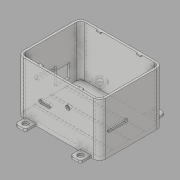
# Autodesk Inventor part: DispenserElectronicsBoxV2
Saved by Autodesk Inventor 2017 (Build 210142000, 142)
## iProperties
Created: 2017-05-31
Part Number: DispenserElectronicsBoxV2
Material: Generic
Document SubType Name: Modeling
Designer: gmarsh
Density: 1 g/cm^3
Appearance: Default
Author: gmarsh
Autodesk Inventor part; units mm, degrees
ref_plane "YZ Plane" through (0, 0, 0) normal (1, 0, 0) x (0, 1, 0)
ref_plane "XZ Plane" through (0, 0, 0) normal (0, 1, 0) x (-1, 0, 0)
ref_plane "XY Plane" through (0, 0, 0) normal (0, 0, 1) x (1, 0, 0)
sketch "Sketch1" plane through (0, 0, 0) normal (0, 0, 1) x (1, 0, 0)
  line L0 (-32.9996, 28) -> (32.9996, 28)
  line L1 (36.9996, 24) -> (36.9996, -24)
  line L2 (32.9996, -28) -> (-32.9996, -28)
  line L3 (-36.9996, -24) -> (-36.9996, 24)
  arc A0 (36.9996, 24) -> (32.9996, 28) centre (32.9996, 24) ccw
  arc A1 (32.9996, -28) -> (36.9996, -24) centre (32.9996, -24) ccw
  arc A2 (-36.9996, -24) -> (-32.9996, -28) centre (-32.9996, -24) ccw
  arc A3 (-32.9996, 28) -> (-36.9996, 24) centre (-32.9996, 24) ccw
  point P0 (0, 0)
  dimension "d0" = 4
  constraints: 8 end point, 8 point on circle, 8 tangent, 4 centre point, 3 equal radius, 2 parallel, 1 horizontal, 1 perpendicular
  measures "d0" radius of A0
surface extrude "ExtrusionSrf1" sketch "Sketch1" along normal blind 50 shown no curves L1 A1 L2 A2 L3 A3 L0 A0
thicken "Thicken1" operation new thickness 2 both sides no extend neighbours no toward (1, 0, 0) faces at (36.9996, 8, 16.6667) (35.7203, -26.9322, 33.3333) (10.9999, -28, 33.3333) (-35.7203, -26.9322, 33.3333) (-36.9996, -8, 16.6667) (-35.9318, 26.7207, 33.3333) (-10.9999, 28, 33.3333) (35.7203, 26.9322, 33.3333)
sketch "Sketch2" plane through (32.9996, -30, 0) normal (0, 0, -1) x (-1, 0, 0)
  line L0 (0, 58) -> (66.081, 58)
  line L1 (70.081, 54) -> (70.081, 6)
  line L2 (66.081, 2) -> (0, 2)
  line L3 (-4, 6) -> (-4, 54)
  arc A0 (70.081, 54) -> (66.081, 58) centre (66.081, 54) ccw
  arc A1 (66.081, 2) -> (70.081, 6) centre (66.081, 6) ccw
  arc A2 (-4, 6) -> (0, 2) centre (0, 6) ccw
  arc A3 (0, 58) -> (-4, 54) centre (0, 54) ccw
  point P0 (32.9996, 30)
  point P1 (31, 30)
  dimension "d5" = 4
  constraints: 8 end point, 8 point on circle, 8 tangent, 4 centre point, 3 equal radius, 2 parallel, 1 horizontal, 1 perpendicular
  measures "d5" radius of A0
extrude "Bottom" add sketch "Sketch2" against normal blind 2
sketch "Sketch9" plane through (32.9996, -30, 0) normal (0, 0, -1) x (-1, 0, 0)
  line L0 (61.976, 69.9481) -> (56.0348, 69.9481)
  line L1 (54.0348, 67.9481) -> (54.0348, -8.1004)
  line L2 (56.0348, -10.1004) -> (61.976, -10.1004)
  line L3 (63.976, -8.1004) -> (63.976, 67.9481)
  line L4 (4, -10.0079) -> (9.9992, -10.0079)
  line L5 (11.9992, -8.0079) -> (11.9992, 67.9122)
  line L6 (9.9992, 69.9122) -> (4, 69.9122)
  line L7 (2, 67.9122) -> (2, -8.0079)
  arc A0 (61.976, -10.1004) -> (63.976, -8.1004) centre (61.976, -8.1004) ccw
  arc A1 (54.0348, -8.1004) -> (56.0348, -10.1004) centre (56.0348, -8.1004) ccw
  arc A2 (63.976, 67.9481) -> (61.976, 69.9481) centre (61.976, 67.9481) ccw
  arc A3 (56.0348, 69.9481) -> (54.0348, 67.9481) centre (56.0348, 67.9481) ccw
  arc A4 (2, -8.0079) -> (4, -10.0079) centre (4, -8.0079) ccw
  arc A5 (9.9992, -10.0079) -> (11.9992, -8.0079) centre (9.9992, -8.0079) ccw
  arc A6 (11.9992, 67.9122) -> (9.9992, 69.9122) centre (9.9992, 67.9122) ccw
  arc A7 (4, 69.9122) -> (2, 67.9122) centre (4, 67.9122) ccw
  point P0 (32.9996, 30)
  point P1 (2, -10.0079)
  point P2 (11.9992, 69.9122)
  dimension "d18" = 2
  constraints: 16 end point, 16 point on circle, 16 tangent, 8 centre point, 7 equal radius, 4 parallel, 4 point on line, 2 horizontal, 2 perpendicular
  measures "d18" radius of A0
extrude "Mounting Tabs" add sketch "Sketch9" against normal blind 2
sketch "Sketch10" plane through (32.9996, -30, 2) normal (0, 0, 1) x (1, 0, 0)
  circle A0 centre (-59, 65) radius 2.5
  circle A1 centre (-7, 65) radius 2.5
  circle A2 centre (-7, -5) radius 2.5
  circle A3 centre (-59, -5) radius 2.5
  point P0 (-32.9996, 30)
  dimension "d21" = 5
  dimension "d22" = 5
  dimension "d23" = 5
  dimension "d24" = 5
  constraints: 4 centre point
  measures "d21" diameter of A0
  measures "d22" diameter of A1
  measures "d23" diameter of A2
  measures "d24" diameter of A3
extrude "Mounting Tab Holes" cut sketch "Sketch10" against normal blind 2
sketch "Sketch4" plane through (38.9996, -24, 0) normal (1, 0, 0) x (0, 0, -1)
  line L0 (-2, 48) -> (-2, 0) projected
  circle A0 centre (-2, 24) radius 1
  circle A1 centre (-2, 8) radius 1
  circle A2 centre (-2, 38) radius 1
  point P0 (0, 24)
  constraints: 3 centre point, 2 point on line, 1 midpoint
extrude "Bottom Ridges" add sketch "Sketch4" against normal blind 76
sketch "Sketch6" plane through (-32.9996, -28, 50) normal (0, 1, 0) x (1, 0, 0)
  line L0 (54, 0) -> (50, 0)
  line L1 (50, 0) -> (50, 1)
  line L2 (50, 1) -> (54, 1)
  line L3 (54, 1) -> (54, 0)
  line L4 (16, 0) -> (12, 0)
  line L5 (12, 0) -> (12, 1)
  line L6 (12, 1) -> (16, 1)
  line L7 (16, 1) -> (16, 0)
  point P0 (32.9996, 50)
  constraints: 16 end point, 4 parallel, 2 horizontal, 2 perpendicular, 2 point on line
extrude "Bottom Latch" add sketch "Sketch6" along normal blind 1
sketch "Sketch8" plane through (-32.9996, 28, 50) normal (0, -1, 0) x (1, 0, 0)
  line L0 (65.9992, 0) -> (0, 0) projected
  line L1 (12, -1) -> (16, -1) projected
  line L2 (12, 0) -> (16, 0)
  line L3 (16, 0) -> (16, -1)
  line L4 (16, -1) -> (12, -1)
  line L5 (12, -1) -> (12, 0)
  line L6 (50, -1) -> (50, 0) projected
  line L7 (54, -1) -> (50, -1) projected
  line L8 (50, 0) -> (54, 0)
  line L9 (54, 0) -> (54, -1)
  line L10 (54, -1) -> (50, -1)
  line L11 (50, -1) -> (50, 0)
  point P0 (32.9996, -50)
  constraints: 16 end point, 4 parallel, 2 horizontal, 2 perpendicular
extrude "Top Latch" add sketch "Sketch8" along normal blind 1
sketch "Sketch11" plane through (-38.9996, -24, 0) normal (-1, 0, 0) x (0, 0, 1)
  line L0 (22, 28) -> (22, 12) construction
  line L1 (20.5, 28) -> (20.5, 12)
  line L2 (23.5, 12) -> (23.5, 28)
  arc A0 (23.5, 28) -> (20.5, 28) centre (22, 28) ccw
  arc A1 (20.5, 12) -> (23.5, 12) centre (22, 12) ccw
  line L3 (20, 29) -> (7.0332, 29)
  line L4 (7.0332, 29) -> (7.0332, 41.9562)
  line L5 (7.0332, 41.9562) -> (20, 41.9562)
  line L6 (20, 41.9562) -> (20, 29)
  line L7 (8, 10) -> (20, 10)
  line L8 (20, 10) -> (20, 0)
  line L9 (20, 0) -> (8, 0)
  line L10 (8, 0) -> (8, 10)
  point P0 (0, 24)
  point P1 (22, 20)
  dimension "d29" = 16
  dimension "d30" = 3
  constraints: 24 end point, 5 parallel, 4 point on circle, 4 tangent, 2 centre point, 2 horizontal, 2 perpendicular, 1 midpoint, 1 vertical
  measures "d29" distance of L0.start L0.end
  measures "d30" diameter of A1
extrude "R Holes" cut sketch "Sketch11" against normal blind 2 contours A0 L2 A1 L1 | L3 L4 L5 L6
sketch "Sketch12" plane through (38.9996, -24, 0) normal (1, 0, 0) x (0, 0, -1)
  line L0 (-22, 3) -> (-22, 19) construction
  line L1 (-20.5, 3) -> (-20.5, 19)
  line L2 (-23.5, 19) -> (-23.5, 3)
  arc A0 (-23.5, 3) -> (-20.5, 3) centre (-22, 3) ccw
  arc A1 (-20.5, 19) -> (-23.5, 19) centre (-22, 19) ccw
  point P0 (0, 24)
  point P1 (-22, 11)
  dimension "d31" = 16
  dimension "d32" = 3
  constraints: 8 end point, 4 point on circle, 4 tangent, 2 centre point, 1 midpoint, 1 parallel, 1 vertical
  measures "d31" distance of L0.start L0.end
  measures "d32" diameter of A1
extrude "L Holes" cut sketch "Sketch12" against normal blind 2
sketch "Sketch13" plane through (-32.9996, -30, 50) normal (0, -1, 0) x (1, 0, 0)
  line L0 (16, -28) -> (24, -28) construction
  line L1 (16, -29.5) -> (24, -29.5)
  line L2 (24, -26.5) -> (16, -26.5)
  arc A0 (16, -26.5) -> (16, -29.5) centre (16, -28) ccw
  arc A1 (24, -29.5) -> (24, -26.5) centre (24, -28) ccw
  line L3 (38, -30) -> (46, -30) construction
  line L4 (38, -31.5) -> (46, -31.5)
  line L5 (46, -28.5) -> (38, -28.5)
  arc A2 (38, -28.5) -> (38, -31.5) centre (38, -30) ccw
  arc A3 (46, -31.5) -> (46, -28.5) centre (46, -30) ccw
  circle A4 centre (42, -20) radius 2
  point P0 (32.9996, -50)
  point P1 (20, -28)
  point P2 (42, -30)
  dimension "d35" = 8
  dimension "d36" = 3
  dimension "d42" = 3
  constraints: 16 end point, 8 point on circle, 5 centre point, 4 tangent, 2 midpoint, 1 horizontal, 1 parallel
  measures "d35" distance of L0.start L0.end
  measures "d36" diameter of A1
  measures "d42" diameter of A3
extrude "Top Holes" cut sketch "Sketch13" against normal blind 2 contours A0 L2 A1 L1 | A4
body "Solid1"
body "Srf1"
